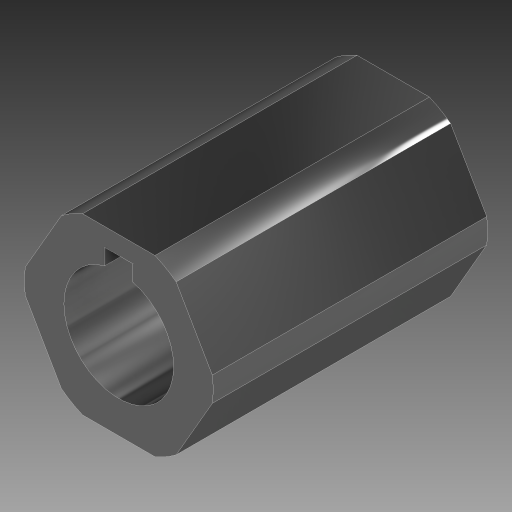
# Autodesk Inventor part: 8mm to 500 Hex Adapter
Saved by Autodesk Inventor 2023 (Build 270158030, 158C)
## iProperties
Created: 2023-01-27
Part Number: 8mm to 500 Hex Adapter
Material: Aluminum 7075
Document SubType Name: Modeling
Designer: Max Boord
Density: 2.7 g/cm^3
Appearance: Glazed - Black
Density: 2.81 g/cm^3
Author: Max Boord
Autodesk Inventor part; units mm, degrees
ref_plane "YZ Plane" through (0, 0, 0) normal (1, 0, 0) x (0, 1, 0)
ref_plane "XZ Plane" through (0, 0, 0) normal (0, 1, 0) x (-1, 0, 0)
ref_plane "XY Plane" through (0, 0, 0) normal (0, 0, 1) x (1, 0, 0)
sketch "Sketch1" plane through (0, 0, 0) normal (0, 0, 1) x (1, 0, 0)
  line L0 (-6.8168, 0.893) -> (-4.1818, 5.457)
  line L1 (-2.635, 6.35) -> (2.635, 6.35)
  line L2 (4.1818, 5.457) -> (6.8168, 0.893)
  line L3 (6.8168, -0.893) -> (4.1818, -5.457)
  line L4 (2.635, -6.35) -> (-2.635, -6.35)
  line L5 (-4.1818, -5.457) -> (-6.8168, -0.893)
  circle A0 centre (0, 0) radius 4
  line L6 (-1.035, 3.8638) -> (-1.035, 5.0258)
  line L7 (-1.035, 5.0258) -> (1.035, 5.0258)
  line L8 (1.035, 5.0258) -> (1.035, 3.8638)
  arc A1 (4.1818, 5.457) -> (2.635, 6.35) centre (0, 0) ccw
  arc A2 (6.8168, -0.893) -> (6.8168, 0.893) centre (0, 0) ccw
  arc A3 (2.635, -6.35) -> (4.1818, -5.457) centre (0, 0) ccw
  arc A4 (-4.1818, -5.457) -> (-2.635, -6.35) centre (0, 0) ccw
  arc A5 (-2.635, 6.35) -> (-4.1818, 5.457) centre (0, 0) ccw
  arc A6 (-6.8168, 0.893) -> (-6.8168, -0.893) centre (0, 0) ccw
  point P0 (0, 5.0258)
  dimension "d0" = 12.7
  dimension "d1" = 8
  dimension "d2" = 2.07
  dimension "d4" = 1.162
  dimension "d6" = 13.75
  constraints: 18 end point, 14 point on circle, 7 centre point, 5 concentric, 3 coincident, 2 perpendicular, 1 horizontal, 1 midpoint, 1 vertical, 1 vertical alignment, 7 other
  measures "d0" distance between parallel lines of L4 L1
  measures "d1" diameter of A0
  measures "d2" distance of L6.end L7.end
  measures "d4" distance of L6.start L6.end
  measures "d6" diameter of A6
extrude "Extrusion1" add sketch "Sketch1" along normal mid plane 20
delete_face "Delete Face1" [suppressed]
body "Solid1"
